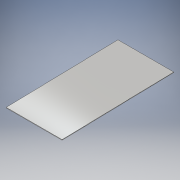
# Autodesk Inventor part: Roof
Saved by Autodesk Inventor 2017 (Build 210142000, 142)
## iProperties
Created: 2021-04-11
Part Number: Roof
Material: Aluminum 6061-AHC
Document SubType Name: Modeling
Designer: udays
Density: 2.7 g/cm^3
Appearance: Aluminum - Dark
Author: udays
Autodesk Inventor part; units mm, degrees
ref_plane "YZ Plane" through (0, 0, 0) normal (1, 0, 0) x (0, 1, 0)
ref_plane "XZ Plane" through (0, 0, 0) normal (0, 1, 0) x (-1, 0, 0)
ref_plane "XY Plane" through (0, 0, 0) normal (0, 0, 1) x (1, 0, 0)
sketch "Sketch1" plane through (0, 0, 0) normal (1, 0, 0) x (0, 1, 0)
  line L0 (0, 0) -> (177.8, 0) construction
  line L1 (177.8, 0) -> (177.8, -5130.8) construction
  line L2 (177.8, -5130.8) -> (304.8, -5130.8) construction
  line L3 (177.8, 0) -> (304.8, -5130.8)
  line L4 (177.8, 0) -> (203.2, 0)
  line L5 (203.2, 0) -> (325.4055, -5130.3067)
  line L6 (304.8, -5130.8) -> (325.4172, -5130.8)
  line L7 (304.8, -5130.8) -> (325.4172, -5130.8) construction
  line L8 (325.4172, -5130.8) -> (325.4055, -5130.3067)
  dimension "d0" = 177.8
  dimension "d1" = 5130.8
  dimension "d2" = 127
  dimension "d3" = 25.4
  dimension "d4" = 0
  constraints: 18 end point, 4 horizontal, 2 collinear, 1 vertical
  measures "d0" distance of L0.start L0.end
  measures "d1" distance of L0.end L1.end
  measures "d2" distance of L1.end L2.end
  measures "d3" distance of L0.end L4.end
  measures "d4" distance between parallel lines of L6 L7
extrude "Extrusion1" add sketch "Sketch1" along normal blind 2565.4
sketch "Sketch2" plane through (0, 304.8, -5130.8) normal (0, -0.9996938, -0.0247449) x (1, 0, 0)
  line L0 (0, 5131.743) -> (2565.4, 5131.743) construction
  line L1 (1282.7, 5131.743) -> (1282.7, 0) construction
  line L2 (0, 0) -> (2565.4, 0) construction
  line L3 (2565.4, 5132.3715) -> (2565.4, 0) construction
  line L4 (2565.4, 2566.1858) -> (0, 2566.1858) construction
  line L5 (1282.7, 5131.743) -> (1282.7, 4621.1725) construction
  line L6 (1282.7, 4621.1725) -> (1282.7, 4110.6021) construction
  line L7 (1282.7, 4110.6021) -> (1282.7, 3600.0316) construction
  line L8 (1282.7, 3600.0316) -> (1282.7, 3089.4611) construction
  line L9 (1282.7, 3089.4611) -> (1282.7, 2566.1858) construction
  line L10 (0, 4646.5725) -> (2565.4, 4646.5725)
  line L11 (2565.4, 4646.5725) -> (2565.4, 4595.7725)
  line L12 (2565.4, 4595.7725) -> (0, 4595.7725)
  line L13 (0, 4595.7725) -> (0, 4646.5725)
  line L14 (0, 4646.5725) -> (2565.4, 4595.7725) construction
  line L15 (2565.4, 4646.5725) -> (0, 4595.7725) construction
  line L16 (0, 4136.0021) -> (2565.4, 4136.0021)
  line L17 (2565.4, 4136.0021) -> (2565.4, 4085.2021)
  line L18 (2565.4, 4085.2021) -> (0, 4085.2021)
  line L19 (0, 4085.2021) -> (0, 4136.0021)
  line L20 (0, 4136.0021) -> (2565.4, 4085.2021) construction
  line L21 (2565.4, 4136.0021) -> (0, 4085.2021) construction
  line L22 (0, 3625.4316) -> (2565.4, 3625.4316)
  line L23 (2565.4, 3625.4316) -> (2565.4, 3574.6316)
  line L24 (2565.4, 3574.6316) -> (0, 3574.6316)
  line L25 (0, 3574.6316) -> (0, 3625.4316)
  line L26 (0, 3625.4316) -> (2565.4, 3574.6316) construction
  line L27 (2565.4, 3625.4316) -> (0, 3574.6316) construction
  line L28 (0, 3114.8611) -> (2565.4, 3114.8611)
  line L29 (2565.4, 3114.8611) -> (2565.4, 3064.0611)
  line L30 (2565.4, 3064.0611) -> (0, 3064.0611)
  line L31 (0, 3064.0611) -> (0, 3114.8611)
  line L32 (0, 3114.8611) -> (2565.4, 3064.0611) construction
  line L33 (2565.4, 3114.8611) -> (0, 3064.0611) construction
  line L34 (0, 5132.3715) -> (0, 0) projected
  line L35 (2565.4, 2566.1858) -> (0, 2566.1858)
  line L36 (0, 2566.1858) -> (0, 2591.5858)
  line L37 (0, 2591.5858) -> (2565.4, 2591.5858)
  line L38 (2565.4, 2591.5858) -> (2565.4, 2566.1858)
  point P0 (0, 5136.7712)
  dimension "d7" = 510.5705
  dimension "d8" = 510.5705
  dimension "d9" = 510.5705
  dimension "d10" = 510.5705
  dimension "d11" = 50.8
  dimension "d12" = 50.8
  dimension "d13" = 50.8
  dimension "d14" = 2565.4
  dimension "d15" = 50.8
  dimension "d16" = 25.4
  constraints: 70 end point, 13 midpoint, 10 parallel, 8 point on line, 6 horizontal, 6 perpendicular, 1 collinear
  measures "d7" distance of L5.start L5.end
  measures "d8" distance of L5.end L6.end
  measures "d9" distance of L6.end L7.end
  measures "d10" distance of L7.end L8.end
  measures "d11" distance of L10.end L11.end
  measures "d12" distance of L16.end L17.end
  measures "d13" distance of L22.end L23.end
  measures "d14" distance of L29.end L30.end
  measures "d15" distance of L28.end L29.end
  measures "d16" distance of L35.end L36.end
extrude "Extrusion2" cut sketch "Sketch2" against normal blind 6.35
sketch "Sketch3" plane through (0, 304.8, -5130.8) normal (0, -0.9996938, -0.0247449) x (1, 0, 0)
  line L0 (2565.4, 2566.1858) -> (0, 2566.1858) construction
  line L1 (2565.4, 2566.1858) -> (0, 2565.6164) construction
  line L2 (0, -0.5102) -> (0, 5131.743) construction
  point P0 (0, 5136.7712)
  constraints: 2 end point, 1 midpoint
mirror "Mirror1" about plane through (2565.4, 241.3, -2565.4) normal (0, -0.0247449, 0.9996938) of "Extrusion2"
body "Solid1"
